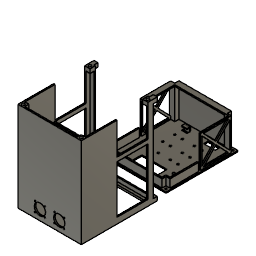
all 600 w (Autodesk Fusion 360 design; units mm, degrees)
part number: 2026-06-05-11-29-00-149
Autodesk Fusion 360 part; units mm, degrees
note: some values were not read from the file. Set by a fixed rule: which sketch regions a step uses.
(part 1 of 2)
sketch "Sketch3" plane through (0, 0, 0) normal (0, 0, 1) x (1, 0, 0)
  line L0 (79.125, -47) -> (-79.125, -47)
  line L1 (-79.125, -47) -> (-79.125, 47)
  line L2 (-79.125, 47) -> (79.125, 47)
  line L3 (79.125, 47) -> (79.125, -47)
  line L4 (79.125, -47) -> (-79.125, 47) construction
  line L5 (-79.125, -47) -> (79.125, 47) construction
  dimension "d3" = 94
  dimension "d4" = 158.25
  constraint horizontal L0
  constraint perpendicular L0 L1
  constraint parallel L0 L2
  constraint parallel L1 L3
  constraint coincident L4 origin
  constraint coincident L5 origin
  measures "d3" distance of L0.end L1.end
  measures "d4" distance of L1.end L2.end
extrude "Extrude1" add sketch "Sketch3" along normal blind 15 makes body 1
sketch "Sketch4" plane through (0, 0, 15) normal (0, 0, 1) x (-1, 0, 0)
  line L0 (-79.125, -47) -> (79.125, -47)
  line L1 (79.125, -47) -> (79.125, 47)
  line L2 (79.125, 47) -> (-79.125, 47)
  line L3 (-79.125, 47) -> (-79.125, -47)
  line L4 (-75.625, 43.5) -> (75.625, 43.5)
  line L5 (75.625, 43.5) -> (75.625, -43.5)
  line L6 (75.625, -43.5) -> (-75.625, -43.5)
  line L7 (-75.625, -43.5) -> (-75.625, 43.5)
  dimension "d7" = 3.5
  dimension "d9" = 3.5
  dimension "d10" = 3.5
  dimension "d11" = 3.5
  constraint horizontal L4
  constraint perpendicular L4 L5
  constraint parallel L4 L6
  constraint parallel L5 L7
  measures "d7" distance of L2 L4
  measures "d9" distance of L3 L7
  measures "d10" distance of L1 L5
  measures "d11" distance of L0 L6
extrude "Extrude2" cut sketch "Sketch4" against normal blind 10 contours L4 L5 L6 L7 bodies 1
sketch "Sketch5" plane through (0, 0, 5) normal (0, 0, 1) x (-1, 0, 0)
  line L0 (-75.625, -43.5) -> (75.625, -43.5)
  line L1 (75.625, -43.5) -> (75.625, 43.5)
  line L2 (75.625, 43.5) -> (-75.625, 43.5)
  line L3 (-75.625, 43.5) -> (-75.625, -43.5)
  line L4 (-69.125, 37) -> (69.125, 37)
  line L5 (69.125, 37) -> (69.125, -37)
  line L6 (69.125, -37) -> (-69.125, -37)
  line L7 (-69.125, -37) -> (-69.125, 37)
  dimension "d14" = 6.5
  dimension "d15" = 6.5
  dimension "d16" = 6.5
  dimension "d17" = 6.5
  constraint horizontal L4
  constraint perpendicular L4 L5
  constraint parallel L4 L6
  constraint parallel L5 L7
  measures "d14" distance of L3 L7
  measures "d15" distance of L2 L4
  measures "d16" distance of L0 L6
  measures "d17" distance of L1 L5
extrude "Extrude3" cut sketch "Sketch5" against normal blind 5 contours L4 L5 L6 L7 bodies 1
sketch "Sketch6" plane through (0, -47, 0) normal (0, -1, 0) x (1, 0, 0)
  line L0 (-79.125, 0) -> (79.125, 0)
  line L1 (79.125, 0) -> (79.125, 15)
  line L2 (79.125, 15) -> (-79.125, 15)
  line L3 (-79.125, 15) -> (-79.125, 0)
  line L4 (-79.125, 5) -> (79.125, 5)
  line L5 (79.125, 5) -> (79.125, 0)
  line L6 (79.125, 0) -> (-79.125, 0)
  line L7 (-79.125, 0) -> (-79.125, 5)
  dimension "d20" = 5
  constraint horizontal L4
  constraint vertical L5
  constraint horizontal L6
  constraint vertical L7
  constraint coincident L0.end L1.start
  constraint coincident L3 L4.start
  measures "d20" distance of L4 L6
extrude "Extrude4" add sketch "Sketch6" along normal blind 86 contours L0 L1 L3 L4 L5 L6 L7 bodies 1
sketch "Sketch7" plane through (0, 0, 5) normal (0, 0, 1) x (-1, 0, 0)
  line L0 (-79.125, 47) -> (79.125, 47)
  line L1 (79.125, 47) -> (79.125, 133)
  line L2 (79.125, 133) -> (-79.125, 133)
  line L3 (-79.125, 133) -> (-79.125, 47)
  line L4 (79.125, 47) -> (75.625, 47)
  line L5 (75.625, 47) -> (75.625, 129.5)
  line L6 (75.625, 133) -> (79.125, 133)
  line L7 (79.125, 133) -> (79.125, 47)
  line L8 (79.125, 133) -> (-79.125, 133)
  line L9 (-79.125, 133) -> (-79.125, 118.5)
  line L10 (-75.625, 129.5) -> (75.625, 129.5)
  line L11 (79.125, 118.5) -> (79.125, 133)
  line L12 (-79.125, 133) -> (-75.625, 133)
  line L13 (-75.625, 129.5) -> (-75.625, 47)
  line L14 (-75.625, 47) -> (-79.125, 47)
  line L15 (-79.125, 47) -> (-79.125, 133)
  dimension "d23" = 3.5
  dimension "d24" = 3.5
  dimension "d25" = 3.5
  constraint horizontal L4
  constraint vertical L5
  constraint horizontal L6
  constraint vertical L7
  constraint coincident L2 L6.start
  constraint coincident L0.end L1.start
  constraint horizontal L8
  constraint vertical L9
  constraint horizontal L10
  constraint vertical L11
  constraint coincident L3 L9.end
  constraint coincident L1.end L2.start
  constraint horizontal L12
  constraint vertical L13
  constraint horizontal L14
  constraint vertical L15
  constraint coincident L0 L13.end
  measures "d23" distance of L5 L7
  measures "d24" distance of L8 L10
  measures "d25" distance of L13 L15
extrude "Extrude5" add sketch "Sketch7" along normal blind 10 contours L0 L1 L2 L3 L4 L5 L6 L7 L8 L9 L10 L11 L12 L13 L14 L15 bodies 1
sketch "Sketch8" plane through (0, 0, 15) normal (0, 0, 1) x (-1, 0, 0)
  line L0 (75.625, 47) -> (-75.625, 47)
  line L1 (-75.625, 47) -> (-75.625, 129.5)
  line L2 (-75.625, 129.5) -> (75.625, 129.5)
  line L3 (75.625, 129.5) -> (75.625, 47)
  line L4 (75.625, 43.5) -> (75.625, -43.5)
  line L5 (75.625, -43.5) -> (-75.625, -43.5)
  line L6 (-75.625, -43.5) -> (-75.625, 43.5)
  line L7 (-75.625, 43.5) -> (75.625, 43.5)
  line L8 (79.125, -47) -> (79.125, 133)
  line L9 (79.125, 133) -> (-79.125, 133)
  line L10 (-79.125, 133) -> (-79.125, -47)
  line L11 (-79.125, -47) -> (79.125, -47)
  line L12 (75.625, 43.5) -> (79.125, 43.5)
  line L13 (-75.625, 43.5) -> (-79.125, 43.5)
  constraint coincident L4.start L7.end
  constraint coincident L8 L12.end
  constraint perpendicular L8 L12
  constraint coincident L6.end L7.start
  constraint coincident L10 L13.end
  constraint perpendicular L10 L13
extrude "Extrude6" add sketch "Sketch8" along normal blind 130 contours L7 L8 L9 L10 L12 L13 bodies 1
sketch "Sketch9" plane through (0, 0, 15) normal (0, 0, 1) x (-1, 0, 0)
  line L0 (79.125, 43.5) -> (75.625, 43.5)
  line L1 (75.625, 43.5) -> (75.625, -43.5)
  line L2 (75.625, -43.5) -> (-75.625, -43.5)
  line L3 (-75.625, -43.5) -> (-75.625, 43.5)
  line L4 (-75.625, 43.5) -> (-79.125, 43.5)
  line L5 (-79.125, 43.5) -> (-79.125, -47)
  line L6 (-79.125, -47) -> (79.125, -47)
  line L7 (79.125, -47) -> (79.125, 43.5)
  line L8 (-79.125, -47) -> (-75.625, -47)
  line L9 (-75.625, -47) -> (-75.625, -43.5)
  line L10 (-75.625, -43.5) -> (-79.125, -43.5)
  line L11 (-79.125, -43.5) -> (-79.125, -47)
  line L12 (75.625, -43.5) -> (79.125, -43.5)
  line L13 (79.125, -43.5) -> (79.125, -47)
  line L14 (79.125, -47) -> (75.625, -47)
  line L15 (75.625, -47) -> (75.625, -43.5)
  constraint horizontal L8
  constraint vertical L9
  constraint horizontal L10
  constraint vertical L11
  constraint coincident L2.end L3.start
  constraint coincident L5.end L6.start
  constraint horizontal L12
  constraint vertical L13
  constraint horizontal L14
  constraint vertical L15
  constraint coincident L6.end L7.start
  constraint coincident L1.end L2.start
extrude "Extrude7" add sketch "Sketch9" along normal blind 130 contours L6 L7 L12 L13 L14 L15 | L5 L6 L8 L9 L10 L11 bodies 1
extrude "Extrude8" add 1 faces at (75.625, 45.8333, 58.3333) along direction (-1, 0, 0) blind 10 on bodies 1 bodies 1
extrude "Extrude9" add 1 faces at (-75.625, 45.8333, 58.3333) along direction (1, 0, 0) blind 10 on bodies 1 bodies 1
sketch "Sketch10" plane through (0, 43.5, 0) normal (0, -1, 0) x (1, 0, 0)
  line L0 (-79.125, 15) -> (-75.625, 15)
  line L1 (-75.625, 15) -> (-75.625, 5)
  line L2 (-75.625, 5) -> (75.625, 5)
  line L3 (75.625, 5) -> (75.625, 15)
  line L4 (75.625, 15) -> (79.125, 15)
  line L5 (79.125, 15) -> (79.125, 145)
  line L6 (79.125, 145) -> (65.625, 145)
  line L7 (65.625, 145) -> (65.625, 15)
  line L8 (65.625, 15) -> (-65.625, 15)
  line L9 (-65.625, 15) -> (-65.625, 145)
  line L10 (-65.625, 145) -> (-79.125, 145)
  line L11 (-79.125, 145) -> (-79.125, 15)
  line L12 (-79.125, 145) -> (-75.625, 145)
  line L13 (-75.625, 145) -> (-75.625, 15)
  line L14 (-75.625, 15) -> (-79.125, 15)
  line L15 (-79.125, 15) -> (-79.125, 145)
  dimension "d36" = 3.5
  dimension "d37" = 130
  constraint horizontal L12
  constraint vertical L13
  constraint horizontal L14
  constraint vertical L15
  constraint coincident L10.end L11.start
  measures "d36" distance of L10.end L12.end
  measures "d37" distance of L10.end L0.start
extrude "Extrude10" add sketch "Sketch10" along normal blind 10 contours L0 L10 L11 L12 L13 L14 L15 bodies 1
sketch "Sketch11" plane through (0, 43.5, 0) normal (0, -1, 0) x (1, 0, 0)
  line L0 (-75.625, 145) -> (-75.625, 5)
  line L1 (-75.625, 5) -> (75.625, 5)
  line L2 (75.625, 5) -> (75.625, 15)
  line L3 (75.625, 15) -> (79.125, 15)
  line L4 (79.125, 15) -> (79.125, 145)
  line L5 (79.125, 145) -> (65.625, 145)
  line L6 (65.625, 145) -> (65.625, 15)
  line L7 (65.625, 15) -> (-65.625, 15)
  line L8 (-65.625, 15) -> (-65.625, 145)
  line L9 (-65.625, 145) -> (-75.625, 145)
  line L10 (79.125, 15) -> (75.625, 15)
  line L11 (75.625, 15) -> (75.625, 145)
  line L12 (75.625, 145) -> (79.125, 145)
  line L13 (79.125, 145) -> (79.125, 15)
  constraint perpendicular L10 L11
  constraint parallel L10 L12
  constraint parallel L11 L13
  constraint coincident L2.end L3.start
  constraint perpendicular L2 L10
  constraint coincident L3.end L4.start
extrude "Extrude11" add sketch "Sketch11" along normal blind 10 contours L3 L4 L5 L10 L11 L12 L13 bodies 1
sketch "Sketch13" plane through (0, 33.5, 0) normal (0, -1, 0) x (1, 0, 0)
  line L0 (-79.125, 15) -> (-75.625, 15)
  line L1 (-75.625, 15) -> (-75.625, 145)
  line L2 (-75.625, 145) -> (-79.125, 145)
  line L3 (-79.125, 145) -> (-79.125, 15)
  line L4 (-79.125, 145) -> (-75.625, 145)
  line L5 (-75.625, 145) -> (-75.625, 135)
  line L6 (-75.625, 135) -> (-79.125, 135)
  line L7 (-79.125, 135) -> (-79.125, 145)
  dimension "d45" = 10
  constraint horizontal L4
  constraint vertical L5
  constraint horizontal L6
  constraint vertical L7
  constraint coincident L2.end L3.start
  measures "d45" distance of L2.end L6.end
extrude "Extrude13" add sketch "Sketch13" along normal blind 77 contours L1 L2 L3 L4 L5 L6 L7 bodies 1
sketch "Sketch14" plane through (0, 33.5, 0) normal (0, -1, 0) x (1, 0, 0)
  line L0 (79.125, 145) -> (75.625, 145)
  line L1 (75.625, 145) -> (75.625, 15)
  line L2 (75.625, 15) -> (79.125, 15)
  line L3 (79.125, 15) -> (79.125, 145)
  line L4 (75.625, 145) -> (79.125, 145)
  line L5 (79.125, 145) -> (79.125, 135)
  line L6 (79.125, 135) -> (75.625, 135)
  line L7 (75.625, 135) -> (75.625, 145)
  dimension "d48" = 10
  constraint horizontal L4
  constraint vertical L5
  constraint horizontal L6
  constraint vertical L7
  constraint coincident L0.end L1.start
  measures "d48" distance of L0.end L6.end
extrude "Extrude14" add sketch "Sketch14" along normal blind 77 contours L0 L1 L3 L4 L5 L6 L7 bodies 1
sketch "Sketch15" plane through (0, 47, 0) normal (0, 1, 0) x (-1, 0, 0)
  line L0 (65.625, 145) -> (65.625, 15)
  line L1 (65.625, 15) -> (-65.625, 15)
  line L2 (-65.625, 15) -> (-65.625, 145)
  line L3 (79.125, 145) -> (65.625, 145)
  line L4 (-79.125, 145) -> (-79.125, 0)
  line L5 (-79.125, 0) -> (79.125, 0)
  line L6 (79.125, 0) -> (79.125, 145)
  line L7 (79.125, 0) -> (69.125, 0)
  line L8 (69.125, 0) -> (69.125, 10)
  line L9 (69.125, 10) -> (79.125, 10)
  line L10 (79.125, 10) -> (79.125, 0)
  line L11 (-65.625, 145) -> (-79.125, 145)
  dimension "d51" = 10
  dimension "d52" = 10
  constraint horizontal L7
  constraint vertical L8
  constraint horizontal L9
  constraint vertical L10
  constraint coincident L5.end L6.start
  measures "d51" distance of L5.end L7.end
  measures "d52" distance of L5.end L9.end
extrude "Extrude15" add sketch "Sketch15" along normal blind 10 contours L5 L6 L7 L8 L9 L10 bodies 1
sketch "Sketch16" plane through (0, 47, 0) normal (0, 1, 0) x (-1, 0, 0)
  line L0 (69.125, 0) -> (69.125, 10)
  line L1 (69.125, 10) -> (79.125, 10)
  line L2 (79.125, 10) -> (79.125, 145)
  line L3 (79.125, 145) -> (65.625, 145)
  line L4 (-79.125, 145) -> (-79.125, 0)
  line L5 (-79.125, 0) -> (69.125, 0)
  line L6 (65.625, 145) -> (65.625, 15)
  line L7 (65.625, 15) -> (-65.625, 15)
  line L8 (-65.625, 15) -> (-65.625, 145)
  line L9 (-79.125, 0) -> (-69.125, 0)
  line L10 (-69.125, 0) -> (-69.125, 10)
  line L11 (-69.125, 10) -> (-79.125, 10)
  line L12 (-79.125, 10) -> (-79.125, 0)
  line L13 (-65.625, 145) -> (-79.125, 145)
  dimension "d55" = 10
  dimension "d56" = 10
  constraint horizontal L9
  constraint vertical L10
  constraint horizontal L11
  constraint vertical L12
  constraint coincident L4.end L5.start
  measures "d55" distance of L4.end L9.end
  measures "d56" distance of L4.end L11.end
extrude "Extrude16" add sketch "Sketch16" along normal blind 10 contours L4 L5 L9 L10 L11 L12 bodies 1
move_body "Move1" bodies 1 to x (1, 0, 0) y (0, 1, 0) z (0, 0, 1) at (235.1887, 10.9866, 0)
sketch "Sketch18" plane through (0, 0, 0) normal (0, 0, 1) x (1, 0, 0)
  line L0 (79.125, -90) -> (-79.125, -90)
  line L1 (-79.125, -90) -> (-79.125, 90)
  line L2 (-79.125, 90) -> (79.125, 90)
  line L3 (79.125, 90) -> (79.125, -90)
  line L4 (79.125, -90) -> (-79.125, 90) construction
  line L5 (-79.125, -90) -> (79.125, 90) construction
  dimension "d63" = 158.25
  dimension "d64" = 180
  constraint horizontal L0
  constraint perpendicular L0 L1
  constraint parallel L0 L2
  constraint parallel L1 L3
  constraint coincident L4 origin
  constraint coincident L5 origin
  measures "d63" distance of L1.end L2.end
  measures "d64" distance of L0.end L1.end
extrude "Extrude17" add sketch "Sketch18" along normal blind 3 separate body makes body 2
sketch "Sketch19" plane through (0, 0, 3) normal (0, 0, 1) x (-1, 0, 0)
  line L0 (-79.125, -90) -> (79.125, -90)
  line L1 (79.125, -90) -> (79.125, 90)
  line L2 (79.125, 90) -> (-79.125, 90)
  line L3 (-79.125, 90) -> (-79.125, -90)
  line L4 (-31.5, 81) -> (31.5, 81)
  line L5 (31.5, 81) -> (31.5, 40)
  line L6 (31.5, 40) -> (-31.5, 40)
  line L7 (-31.5, 40) -> (-31.5, 81)
  dimension "d67" = 63
  dimension "d68" = 41
  dimension "d329" = 9
  dimension "d367" = 47.625
  constraint horizontal L4
  constraint vertical L5
  constraint horizontal L6
  constraint vertical L7
  measures "d67" distance of L4.start L4.end
  measures "d68" distance of L4.start L6.end
  measures "d329" distance of L2 L4
  measures "d367" distance of L3 L7
extrude "Extrude18" cut sketch "Sketch19" against normal blind 3 contours L4 L5 L6 L7 bodies 2
sketch "Sketch20" plane through (0, 0, 3) normal (0, 0, 1) x (-1, 0, 0)
  line L0 (31.5, 81) -> (31.5, 40)
  line L1 (31.5, 40) -> (-31.5, 40)
  line L2 (-31.5, 40) -> (-31.5, 81)
  line L3 (-31.5, 81) -> (31.5, 81)
  line L4 (-79.125, -90) -> (79.125, -90)
  line L5 (79.125, -90) -> (79.125, 90)
  line L6 (79.125, 90) -> (-79.125, 90)
  line L7 (-79.125, 90) -> (-79.125, -90)
  circle A0 centre (-15, 15) radius 2.5
  circle A1 centre (-34, 15) radius 2.5
  circle A2 centre (-34, -15) radius 2.5
  circle A3 centre (-15, -15) radius 2.5
  circle A4 centre (-15, -45) radius 2.5
  circle A5 centre (-34, -45) radius 2.5
  line L8 (-34, 15) -> (-15, 15)
  line L9 (-15, 15) -> (-15, -15)
  line L10 (-15, -15) -> (-34, -15)
  line L11 (-34, -15) -> (-34, 15)
  line L12 (-15, -45) -> (-15, -15)
  line L13 (-15, -45) -> (-34, -45)
  line L14 (-34, -15) -> (-34, -45)
  circle A6 centre (15, 15) radius 2.5
  circle A7 centre (34, 15) radius 2.5
  circle A8 centre (15, -15) radius 2.5
  circle A9 centre (34, -15) radius 2.5
  circle A10 centre (15, -45) radius 2.5
  circle A11 centre (34, -45) radius 2.5
  line L15 (15, 15) -> (34, 15)
  line L16 (34, 15) -> (34, -15)
  line L17 (34, -15) -> (15, -15)
  line L18 (15, -15) -> (15, 15)
  line L19 (15, -15) -> (15, -45)
  line L20 (15, -45) -> (34, -45)
  line L21 (34, -45) -> (34, -15)
  line L22 (15, 15) -> (-15, 15)
  line L23 (-15, -15) -> (15, -15)
  line L24 (15, -45) -> (-15, -45)
  dimension "d71" = 5
  dimension "d72" = 5
  dimension "d73" = 5
  dimension "d74" = 5
  dimension "d75" = 5
  dimension "d76" = 5
  dimension "d77" = 19
  dimension "d78" = 75
  dimension "d79" = 75
  dimension "d80" = 30
  dimension "d353" = 5
  dimension "d354" = 5
  dimension "d355" = 5
  dimension "d356" = 5
  dimension "d357" = 5
  dimension "d358" = 5
  dimension "d359" = 30
  dimension "d360" = 30
  dimension "d361" = 19
  dimension "d362" = 30
  dimension "d363" = 30
  dimension "d364" = 75
  dimension "d365" = 30
  dimension "d366" = 45.125
  constraint coincident A1.centre L8.start
  constraint coincident A0.centre L8.end
  constraint coincident A3.centre L9.end
  constraint coincident A2.centre L10.end
  constraint coincident A5.centre L13.end
  constraint coincident A4.centre L12.start
  constraint parallel L8 L10
  constraint parallel L10 L13
  constraint equal L8 L10
  constraint equal L10 L13
  constraint equal L11 L12
  constraint perpendicular L10 L11
  constraint perpendicular L10 L14
  constraint coincident A6.centre L15.start
  constraint coincident A7.centre L15.end
  constraint coincident A9.centre L16.end
  constraint coincident A8.centre L17.end
  constraint vertical L18
  constraint coincident A10.centre L19.end
  constraint coincident A11.centre L20.end
  constraint parallel L6 L15
  constraint equal L15 L17
  constraint equal L17 L20
  constraint perpendicular L17 L19
  measures "d71" diameter of A0
  measures "d72" diameter of A1
  measures "d73" diameter of A2
  measures "d74" diameter of A3
  measures "d75" diameter of A4
  measures "d76" diameter of A5
  measures "d77" horizontal distance of A0.centre A1.centre
  measures "d78" distance of L6 A1.centre
  measures "d79" distance of L6 A0.centre
  measures "d80" distance of A1.centre A2.centre
  measures "d353" diameter of A6
  measures "d354" diameter of A7
  measures "d355" diameter of A8
  measures "d356" diameter of A9
  measures "d358" diameter of A11
  measures "d359" vertical distance of A8.centre A10.centre
  measures "d360" distance of A6.centre A8.centre
  measures "d361" horizontal distance of A6.centre A7.centre
  measures "d362" vertical distance of A7.centre A9.centre
  measures "d363" vertical distance of A9.centre A11.centre
  measures "d364" distance of L6 A6.centre
  measures "d365" distance of A0.centre A6.centre
  measures "d366" distance of L7 L11
extrude "Extrude19" cut sketch "Sketch20" against normal blind 3 contours A0 L8 L22 | A0 L9 L22 | A0 L8 L9 | A6 L18 L22 | A6 L15 L22 | A1 L8 L11 | A1 L8 L11 | A3 L9 L10 | A3 L9 L23 | A6 L15 L18 | A3 L12 L23 | A3 L10 L12 | A7 L15 L16 | A7 L15 L16 | A8 L18 L23 | A8 L17 L18 | A2 L11 L14 | A2 L10 L11 | A8 L19 L23 | A2 L10 L14 | A8 L17 L19 | A4 L12 L13 | A4 L12 L24 | A9 L16 L17 | A9 L16 L21 | A9 L17 L21 | A5 L13 L14 | A5 L13 L14 | A4 L13 L24 | A10 L19 L24 | A10 L19 L20 | A10 L20 L24 | A11 L20 L21 | A11 L20 L21 bodies 2
sketch "Sketch21" plane through (0, 0, 3) normal (0, 0, 1) x (-1, 0, 0)
  line L0 (-79.125, -90) -> (79.125, -90)
  line L1 (79.125, -90) -> (79.125, 90)
  line L2 (79.125, 90) -> (-79.125, 90)
  line L3 (-79.125, 90) -> (-79.125, -90)
  line L4 (31.5, 81) -> (31.5, 40)
  line L5 (31.5, 40) -> (-31.5, 40)
  line L6 (-31.5, 40) -> (-31.5, 81)
  line L7 (-31.5, 81) -> (31.5, 81)
  circle A0 centre (-15, -45) radius 2.5
  circle A1 centre (-15, 15) radius 2.5
  circle A2 centre (-15, -15) radius 2.5
  circle A3 centre (-34, -45) radius 2.5
  circle A4 centre (-34, 15) radius 2.5
  circle A5 centre (-34, -15) radius 2.5
  circle A6 centre (49.125, 40) radius 3.5
  circle A7 centre (34, -45) radius 2.5
  circle A8 centre (15, 15) radius 2.5
  circle A9 centre (15, -15) radius 2.5
  circle A10 centre (15, -45) radius 2.5
  circle A11 centre (34, 15) radius 2.5
  circle A12 centre (34, -15) radius 2.5
  dimension "d84" = 7
  dimension "d368" = 50
  dimension "d369" = 30
  measures "d84" diameter of A6
  measures "d368" distance of L2 A6.centre
  measures "d369" distance of L1 A6.centre
extrude "Extrude20" cut sketch "Sketch21" against normal blind 3 contours A6 bodies 2
sketch "Sketch22" plane through (0, 0, 3) normal (0, 0, 1) x (-1, 0, 0)
  circle A0 centre (-34, -15) radius 2.5
  circle A1 centre (-34, -45) radius 2.5
  circle A2 centre (-15, -15) radius 2.5
  circle A3 centre (-15, 15) radius 2.5
  circle A4 centre (-15, -45) radius 2.5
  line L0 (31.5, 81) -> (31.5, 40)
  line L1 (31.5, 40) -> (-31.5, 40)
  line L2 (-31.5, 40) -> (-31.5, 81)
  line L3 (-31.5, 81) -> (31.5, 81)
  line L4 (-79.125, -90) -> (79.125, -90)
  line L5 (79.125, -90) -> (79.125, 90)
  line L6 (79.125, 90) -> (-79.125, 90)
  line L7 (-79.125, 90) -> (-79.125, -90)
  line L8 (21.4933, -61.9167) -> (50.1933, -61.9167)
  line L9 (50.1933, -61.9167) -> (50.1933, -72.9167)
  line L10 (50.1933, -72.9167) -> (21.4933, -72.9167)
  line L11 (21.4933, -72.9167) -> (21.4933, -61.9167)
  circle A5 centre (-34, 15) radius 2.5
  circle A6 centre (34, -15) radius 2.5
  circle A7 centre (34, 15) radius 2.5
  circle A8 centre (15, -45) radius 2.5
  circle A9 centre (15, -15) radius 2.5
  circle A10 centre (15, 15) radius 2.5
  circle A11 centre (34, -45) radius 2.5
  circle A12 centre (49.125, 40) radius 3.5
  dimension "d87" = 28.7
  dimension "d88" = 11
  constraint horizontal L8
  constraint vertical L9
  constraint horizontal L10
  constraint vertical L11
  measures "d87" distance of L8.start L8.end
  measures "d88" distance of L8.start L10.end
extrude "Extrude21" cut sketch "Sketch22" against normal blind 3 contours L8 L9 L10 L11 bodies 2
move_body "Move3" bodies 2 to x (-1, 0, 0) y (0, 1, 0) z (0, 0, -1) at (-44.4015, 0, 3)
sketch "Sketch25" plane through (0, 0, 3) normal (0, 0, 1) x (-1, 0, 0)
  line L0 (-5.7917, -72.9167) -> (-5.7917, -61.9167)
  line L1 (-5.7917, -61.9167) -> (22.9083, -61.9167)
  line L2 (22.9083, -61.9167) -> (22.9083, -72.9167)
  line L3 (22.9083, -72.9167) -> (-5.7917, -72.9167)
  circle A0 centre (78.4015, -15) radius 2.5
  circle A1 centre (78.4015, -45) radius 2.5
  circle A2 centre (59.4015, -15) radius 2.5
  circle A3 centre (59.4015, 15) radius 2.5
  circle A4 centre (59.4015, -45) radius 2.5
  line L4 (12.9015, 40) -> (12.9015, 81)
  line L5 (12.9015, 81) -> (75.9015, 81)
  line L6 (75.9015, 81) -> (75.9015, 40)
  line L7 (75.9015, 40) -> (12.9015, 40)
  line L8 (-34.7235, -90) -> (123.5265, -90)
  line L9 (123.5265, -90) -> (123.5265, 90)
  line L10 (123.5265, 90) -> (-34.7235, 90)
  line L11 (-34.7235, 90) -> (-34.7235, -90)
  line L12 (-21.2235, -87) -> (110.0265, -87)
  line L13 (106.5265, -83.5) -> (-17.7235, -83.5)
  line L14 (116.5265, -73) -> (116.5265, 0)
  line L15 (116.5265, 0) -> (120.0265, 0)
  line L16 (-27.7235, -73) -> (-27.7235, 0)
  line L17 (-27.7235, 0) -> (-31.2235, 0)
  line L18 (-31.2235, 0) -> (-31.2235, -76.5)
  line L19 (-21.2235, -76.5) -> (-31.2235, -76.5)
  line L20 (-17.7235, -76.5) -> (-17.7235, -73)
  line L21 (-17.7235, -73) -> (-27.7235, -73)
  line L22 (-17.7235, -76.5) -> (-17.7235, -83.5)
  line L23 (120.0265, 0) -> (120.0265, -76.5)
  line L24 (110.0265, -76.5) -> (110.0265, -83.5)
  line L25 (110.0265, -83.5) -> (110.0265, -87)
  line L26 (116.5265, -73) -> (106.5265, -73)
  line L27 (106.5265, -83.5) -> (106.5265, -73)
  line L28 (110.0265, -76.5) -> (120.0265, -76.5)
  line L29 (-21.2235, -76.5) -> (-21.2235, -87)
  circle A5 centre (78.4015, 15) radius 2.5
  circle A6 centre (10.4015, -45) radius 2.5
  circle A7 centre (29.4015, 15) radius 2.5
  circle A8 centre (29.4015, -15) radius 2.5
  circle A9 centre (29.4015, -45) radius 2.5
  circle A10 centre (10.4015, 15) radius 2.5
  circle A11 centre (10.4015, -15) radius 2.5
  circle A12 centre (-4.7235, 40) radius 3.5
  dimension "d101" = 3
  dimension "d105" = 3.5
  dimension "d107" = 3.5
  constraint horizontal L12
  constraint horizontal L13
  constraint vertical L14
  constraint horizontal L15
  constraint vertical L16
  constraint horizontal L17
  constraint vertical L18
  constraint horizontal L19
  constraint vertical L20
  constraint horizontal L21
  constraint perpendicular L13 L22
  constraint perpendicular L15 L23
  constraint vertical L24
  constraint perpendicular L26 L27
  constraint perpendicular L23 L28
  constraint perpendicular L19 L29
  measures "d101" distance of L8 L12
  measures "d105" distance of L14.end L15.end
  measures "d107" distance of L16.end L17.end
extrude "Extrude23" add sketch "Sketch25" along normal blind 80 contours L12 L13 L14 L15 L16 L17 L18 L19 L20 L21 L22 L23 L24 L25 L26 L27 L28 L29 bodies 2
sketch "Sketch26" plane through (0, 83.5, 0) normal (0, -1, 0) x (1, 0, 0)
  line L0 (-106.5265, 3) -> (17.7235, 3)
  line L1 (17.7235, 83) -> (-106.5265, 83)
  line L2 (-106.5265, 83) -> (17.7235, 83)
  line L3 (17.7235, 83) -> (17.7235, 79.5)
  line L4 (17.7235, 79.5) -> (-106.5265, 79.5)
  line L5 (-106.5265, 79.5) -> (-106.5265, 83)
  line L6 (17.7235, 3) -> (17.7235, 83)
  line L7 (-106.5265, 83) -> (-106.5265, 3)
  dimension "d108" = 3.5
  dimension "d187" = 124.25
  constraint horizontal L2
  constraint vertical L3
  constraint horizontal L4
  constraint vertical L5
  constraint coincident L1.end L2.start
  measures "d108" distance of L2 L4
  measures "d187" distance of L3 L5
extrude "Extrude24" add sketch "Sketch26" along normal blind 10.5 contours L1 L2 L3 L4 L5 L6 L7 bodies 2
sketch "Sketch27" plane through (-116.5265, 0, 0) normal (1, 0, 0) x (0, 1, 0)
  line L0 (73, 83) -> (0, 83)
  line L1 (0, 83) -> (0, 3)
  line L2 (0, 3) -> (73, 3)
  line L3 (0, 83) -> (73, 83)
  line L4 (73, 83) -> (73, 79.5)
  line L5 (73, 79.5) -> (0, 79.5)
  line L6 (0, 79.5) -> (0, 83)
  line L7 (73, 3) -> (73, 83)
  dimension "d188" = 73
  dimension "d420" = 3.5
  constraint horizontal L3
  constraint vertical L4
  constraint horizontal L5
  constraint vertical L6
  constraint coincident L0.end L1.start
  measures "d188" distance of L0.end L0.start
  measures "d420" distance of L3 L5
extrude "Extrude25" add sketch "Sketch27" along normal blind 10 contours L0 L1 L3 L4 L5 L6 L7 bodies 2
sketch "Sketch30" plane through (0, 0, 145) normal (0, 0, 1) x (-1, 0, 0)
  line L0 (-314.3137, 122.0134) -> (-314.3137, -57.9866)
  line L1 (-314.3137, -57.9866) -> (-300.8137, -57.9866)
  line L2 (-156.0637, -57.9866) -> (-156.0637, 122.0134)
  line L3 (-156.0637, 122.0134) -> (-314.3137, 122.0134)
  line L4 (-310.8137, 118.5134) -> (-159.5637, 118.5134)
  line L5 (-159.5637, 118.5134) -> (-159.5637, 36.0134)
  line L6 (-159.5637, 36.0134) -> (-310.8137, 36.0134)
  line L7 (-310.8137, 36.0134) -> (-310.8137, 118.5134)
  line L8 (-310.8137, -54.4866) -> (-310.8137, 32.5134)
  line L9 (-310.8137, 32.5134) -> (-159.5637, 32.5134)
  line L10 (-159.5637, 32.5134) -> (-159.5637, -54.4866)
  line L11 (-300.8137, -54.4866) -> (-310.8137, -54.4866)
  line L12 (-159.5637, 36.0134) -> (-159.5637, 32.5134)
  line L13 (-159.5637, 32.5134) -> (-156.0637, 32.5134)
  line L14 (-310.8137, 36.0134) -> (-310.8137, 32.5134)
  line L15 (-314.3137, 32.5134) -> (-310.8137, 32.5134)
  line L16 (-300.8137, -57.9866) -> (-300.8137, -54.4866)
  line L17 (-159.5637, -54.4866) -> (-169.5637, -54.4866)
  line L18 (-169.5637, -54.4866) -> (-169.5637, -57.9866)
  line L19 (-169.5637, -57.9866) -> (-156.0637, -57.9866)
  constraint coincident L5.end L6.start
  constraint coincident L9.end L10.start
  constraint coincident L2 L13.end
  constraint perpendicular L2 L13
  constraint coincident L6.end L7.start
  constraint coincident L8.end L9.start
  constraint coincident L0 L15.start
  constraint perpendicular L8 L15
extrude "Extrude27" add sketch "Sketch30" along normal blind 80 contours L0 L2 L3 L4 L5 L7 L12 L13 L14 L15 bodies 1
sketch "Sketch31" plane through (0, 0, 3) normal (0, 0, 1) x (-1, 0, 0)
  line L0 (-34.7235, -90) -> (123.5265, -90)
  line L1 (123.5265, -90) -> (123.5265, 90)
  line L2 (123.5265, 90) -> (-34.7235, 90)
  line L3 (-34.7235, 90) -> (-34.7235, -90)
  line L4 (12.9015, 40) -> (12.9015, 81)
  line L5 (12.9015, 81) -> (75.9015, 81)
  line L6 (75.9015, 81) -> (75.9015, 40)
  line L7 (75.9015, 40) -> (12.9015, 40)
  circle A0 centre (59.4015, -45) radius 2.5
  circle A1 centre (59.4015, 15) radius 2.5
  circle A2 centre (59.4015, -15) radius 2.5
  circle A3 centre (78.4015, -45) radius 2.5
  circle A4 centre (78.4015, -15) radius 2.5
  line L8 (-5.7917, -72.9167) -> (-5.7917, -61.9167)
  line L9 (-5.7917, -61.9167) -> (22.9083, -61.9167)
  line L10 (22.9083, -61.9167) -> (22.9083, -72.9167)
  line L11 (22.9083, -72.9167) -> (-5.7917, -72.9167)
  line L12 (116.5265, -73) -> (116.5265, 0)
  line L13 (116.5265, 0) -> (120.0265, 0)
  line L14 (110.0265, -87) -> (-21.2235, -87)
  line L15 (-31.2235, 0) -> (-27.7235, 0)
  line L16 (-27.7235, 0) -> (-27.7235, -73)
  line L17 (-17.7235, -83.5) -> (106.5265, -83.5)
  line L18 (106.5265, 83) -> (-17.7235, 83)
  line L19 (-27.7235, 73) -> (-27.7235, 5)
  line L20 (-27.7235, 5) -> (-31.2235, 5)
  line L21 (-31.2235, 5) -> (-31.2235, 76.5)
  line L22 (116.5265, 73) -> (116.5265, 5)
  line L23 (120.0265, 5) -> (120.0265, 76.5)
  line L24 (106.5265, -83.5) -> (106.5265, -73)
  line L25 (106.5265, -73) -> (116.5265, -73)
  line L26 (120.0265, 0) -> (120.0265, -76.5)
  line L27 (120.0265, -76.5) -> (110.0265, -76.5)
  line L28 (110.0265, -76.5) -> (110.0265, -87)
  line L29 (-21.2235, -87) -> (-21.2235, -76.5)
  line L30 (-21.2235, -76.5) -> (-31.2235, -76.5)
  line L31 (-31.2235, -76.5) -> (-31.2235, 0)
  line L32 (-27.7235, -73) -> (-17.7235, -73)
  line L33 (-17.7235, -73) -> (-17.7235, -83.5)
  line L34 (110.0265, 76.5) -> (120.0265, 76.5)
  line L35 (106.5265, 83) -> (106.5265, 73)
  line L36 (120.0265, 76.5) -> (110.0265, 76.5)
  line L37 (-21.2235, 86.5) -> (104.0099, 86.5)
  line L38 (116.5265, 73) -> (106.5265, 73)
  line L39 (110.0265, 76.5) -> (110.0265, 86.5)
  line L40 (-21.2235, 86.5) -> (-21.2235, 76.5)
  line L41 (-21.2235, 76.5) -> (-33.7401, 76.5)
  line L42 (-21.2235, 86.5) -> (-17.7235, 86.5)
  line L43 (-21.2235, 76.5) -> (-21.2235, 86.5)
  line L44 (-31.2235, 76.5) -> (-21.2235, 76.5)
  line L45 (-31.2235, 73) -> (-31.2235, 76.5)
  circle A5 centre (78.4015, 15) radius 2.5
  line L46 (-17.7235, 83) -> (-17.7235, 73)
  line L47 (-27.7235, 73) -> (-17.7235, 73)
  line L48 (104.0099, 86.5) -> (110.0265, 86.5)
  circle A6 centre (10.4015, -15) radius 2.5
  circle A7 centre (10.4015, 15) radius 2.5
  circle A8 centre (29.4015, -45) radius 2.5
  circle A9 centre (29.4015, -15) radius 2.5
  circle A10 centre (29.4015, 15) radius 2.5
  circle A11 centre (10.4015, -45) radius 2.5
  circle A12 centre (-4.7235, 40) radius 3.5
  line L49 (120.0265, 5) -> (116.5265, 5)
  dimension "d196" = 3.5
  dimension "d331" = 13.5
  dimension "d332" = 3.5
  dimension "d333" = 13.5
  dimension "d334" = 3.5
  dimension "d337" = 3.5
  dimension "d338" = 3.5
  dimension "d339" = 13.5
  dimension "d340" = 13.5
  dimension "d341" = 3.5
  dimension "d342" = 3.5
  dimension "d344" = 131.25
  dimension "d345" = 3.5
  dimension "d346" = 3.5
  dimension "d347" = 3.5
  dimension "d381" = 5
  dimension "d382" = 5
  constraint vertical L40
  constraint horizontal L41
  constraint horizontal L42
  constraint vertical L43
  constraint horizontal L44
  constraint vertical L45
  constraint perpendicular L46 L47
  constraint perpendicular L39 L48
  constraint perpendicular L22 L49
  measures "d196" distance of L37.start L42.end
  measures "d331" distance of L37 L47
  measures "d332" distance of L41 L47
  measures "d333" distance of L45 L46
  measures "d334" distance of L19 L21
  measures "d337" distance of L18 L37
  measures "d338" distance of L35 L39
  measures "d339" distance of L37 L38
  measures "d340" distance of L23 L35
  measures "d341" distance of L34 L38
  measures "d342" distance of L22 L23
  measures "d344" distance of L39 L40
  measures "d345" distance of L40 L46
  measures "d346" distance of L1 L23
  measures "d347" distance of L2 L37
  measures "d381" distance of L15 L20
  measures "d382" distance of L13 L49
extrude "Extrude28" add sketch "Sketch31" along normal blind 20 contours L18 L19 L20 L21 L22 L23 L34 L35 L36 L37 L38 L39 L40 L41 L42 L43 L44 L45 L46 L47 L48 L49 bodies 2
sketch "Sketch32" plane through (0, 0, 145) normal (0, 0, 1) x (-1, 0, 0)
  line L0 (-156.0637, 32.5134) -> (-159.5637, 32.5134)
  line L1 (-159.5637, 32.5134) -> (-159.5637, -54.4866)
  line L2 (-159.5637, -54.4866) -> (-169.5637, -54.4866)
  line L3 (-310.8137, -54.4866) -> (-310.8137, 32.5134)
  line L4 (-310.8137, 32.5134) -> (-314.3137, 32.5134)
  line L5 (-314.3137, 32.5134) -> (-314.3137, -57.9866)
  line L6 (-169.5637, -57.9866) -> (-156.0637, -57.9866)
  line L7 (-156.0637, -57.9866) -> (-156.0637, 32.5134)
  line L8 (-159.5637, -44.4866) -> (-156.0637, -44.4866)
  line L9 (-169.5637, -54.4866) -> (-169.5637, -57.9866)
  line L10 (-169.5637, -54.4866) -> (-169.5637, -57.9866)
  line L11 (-314.3137, -57.9866) -> (-300.8137, -57.9866)
  line L12 (-300.8137, -57.9866) -> (-300.8137, -54.4866)
  line L13 (-300.8137, -54.4866) -> (-310.8137, -54.4866)
  constraint coincident L1 L8.start
  constraint coincident L7 L8.end
  constraint coincident L2 L9.start
  constraint coincident L6 L9.end
extrude "Extrude31" add sketch "Sketch32" along normal blind 80 contours L1 L2 L6 L7 L8 L9 L10 bodies 1
sketch "Sketch33" plane through (0, 0, 145) normal (0, 0, 1) x (-1, 0, 0)
  line L0 (-310.8137, -54.4866) -> (-310.8137, 32.5134)
  line L1 (-310.8137, -44.4866) -> (-314.3137, -44.4866)
  line L2 (-300.8137, -54.4866) -> (-300.8137, -57.9866)
  line L3 (-300.8137, -54.4866) -> (-310.8137, -54.4866)
  line L4 (-310.8137, 32.5134) -> (-314.3137, 32.5134)
  line L5 (-314.3137, 32.5134) -> (-314.3137, -57.9866)
  line L6 (-314.3137, -57.9866) -> (-300.8137, -57.9866)
  line L7 (-300.8137, -57.9866) -> (-300.8137, -54.4866)
  constraint coincident L0 L1.start
extrude "Extrude30" add sketch "Sketch33" along normal blind 80 contours L0 L1 L2 L3 L5 L6 L7 bodies 1
sketch "Sketch35" plane through (159.5637, 0, 0) normal (1, 0, 0) x (0, 1, 0)
  line L0 (44.4866, 15) -> (-32.5134, 15)
  line L1 (-32.5134, 15) -> (-32.5134, 5)
  line L2 (-32.5134, 5) -> (54.4866, 5)
  line L3 (54.4866, 5) -> (54.4866, 225)
  line L4 (54.4866, 225) -> (44.4866, 225)
  line L5 (44.4866, 225) -> (44.4866, 145)
  line L6 (44.4866, 145) -> (-32.5134, 145)
  line L7 (-32.5134, 145) -> (-32.5134, 135)
  line L8 (-32.5134, 135) -> (44.4866, 135)
  line L9 (44.4866, 135) -> (44.4866, 15)
  line L10 (44.4866, 225) -> (54.4866, 225)
  line L11 (54.4866, 225) -> (54.4866, 215)
  line L12 (54.4866, 215) -> (44.4866, 215)
  line L13 (44.4866, 215) -> (44.4866, 225)
  dimension "d141" = 10
  dimension "d444" = 10
  constraint horizontal L10
  constraint vertical L11
  constraint horizontal L12
  constraint vertical L13
  constraint coincident L4.end L5.start
  measures "d141" distance of L4.end L12.end
  measures "d444" distance of L11 L13
extrude "Extrude32" add sketch "Sketch35" along normal blind 10 contours L3 L4 L5 L10 L11 L12 L13 bodies 1
sketch "Sketch36" plane through (310.8137, 0, 0) normal (-1, 0, 0) x (0, -1, 0)
  line L0 (-54.4866, 225) -> (-54.4866, 5)
  line L1 (-54.4866, 5) -> (32.5134, 5)
  line L2 (32.5134, 5) -> (32.5134, 15)
  line L3 (32.5134, 15) -> (-44.4866, 15)
  line L4 (-44.4866, 15) -> (-44.4866, 135)
  line L5 (-44.4866, 135) -> (32.5134, 135)
  line L6 (32.5134, 135) -> (32.5134, 145)
  line L7 (32.5134, 145) -> (-44.4866, 145)
  line L8 (-44.4866, 145) -> (-44.4866, 225)
  line L9 (-44.4866, 225) -> (-54.4866, 225)
  line L10 (-44.4866, 225) -> (-68.15, 225)
  line L11 (-68.15, 225) -> (-68.15, 215)
  line L12 (-68.15, 215) -> (-44.4866, 215)
  line L13 (-44.4866, 215) -> (-44.4866, 225)
  dimension "d144" = 10
  constraint horizontal L10
  constraint vertical L11
  constraint horizontal L12
  constraint vertical L13
  constraint coincident L8.end L9.start
  measures "d144" distance of L8.end L12.end
extrude "Extrude33" add sketch "Sketch36" along normal blind 10 contours L0 L8 L9 L10 L12 L13 bodies 1
sketch "Sketch37" plane through (0, 57.9866, 0) normal (0, 1, 0) x (-1, 0, 0)
  line L0 (-304.3137, 10) -> (-304.3137, 0)
  line L1 (-304.3137, 0) -> (-166.0637, 0)
  line L2 (-166.0637, 0) -> (-166.0637, 10)
  line L3 (-166.0637, 10) -> (-156.0637, 10)
  line L4 (-156.0637, 10) -> (-156.0637, 225)
  line L5 (-156.0637, 225) -> (-169.5637, 225)
  line L6 (-300.8137, 225) -> (-314.3137, 225)
  line L7 (-314.3137, 225) -> (-314.3137, 10)
  line L8 (-314.3137, 10) -> (-304.3137, 10)
  line L9 (-169.5637, 225) -> (-169.5637, 15)
  line L10 (-169.5637, 15) -> (-300.8137, 15)
  line L11 (-300.8137, 15) -> (-300.8137, 225)
  line L12 (-156.0637, 225) -> (-166.0637, 225)
  line L13 (-166.0637, 225) -> (-166.0637, 215)
  line L14 (-166.0637, 215) -> (-156.0637, 215)
  line L15 (-156.0637, 215) -> (-156.0637, 225)
  dimension "d147" = 10
  dimension "d148" = 10
  constraint horizontal L12
  constraint vertical L13
  constraint horizontal L14
  constraint vertical L15
  constraint coincident L4.end L5.start
  measures "d147" distance of L4.end L12.end
  measures "d148" distance of L4.end L14.end
extrude "Extrude34" add sketch "Sketch37" along normal blind 10 contours L4 L5 L12 L13 L14 L15 bodies 1
sketch "Sketch38" plane through (0, 57.9866, 0) normal (0, 1, 0) x (-1, 0, 0)
  line L0 (-300.8137, 225) -> (-314.3137, 225)
  line L1 (-314.3137, 225) -> (-314.3137, 10)
  line L2 (-314.3137, 10) -> (-304.3137, 10)
  line L3 (-304.3137, 10) -> (-304.3137, 0)
  line L4 (-304.3137, 0) -> (-166.0637, 0)
  line L5 (-166.0637, 0) -> (-166.0637, 10)
  line L6 (-166.0637, 10) -> (-156.0637, 10)
  line L7 (-156.0637, 10) -> (-156.0637, 215)
  line L8 (-156.0637, 215) -> (-166.0637, 215)
  line L9 (-169.5637, 225) -> (-169.5637, 15)
  line L10 (-169.5637, 15) -> (-300.8137, 15)
  line L11 (-300.8137, 15) -> (-300.8137, 225)
  line L12 (-314.3137, 225) -> (-304.3137, 225)
  line L13 (-304.3137, 225) -> (-304.3137, 215)
  line L14 (-304.3137, 215) -> (-314.3137, 215)
  line L15 (-314.3137, 215) -> (-314.3137, 225)
  line L16 (-166.0637, 215) -> (-166.0637, 225)
  line L17 (-166.0637, 225) -> (-169.5637, 225)
  dimension "d151" = 10
  dimension "d443" = 10
  constraint horizontal L12
  constraint vertical L13
  constraint horizontal L14
  constraint vertical L15
  constraint coincident L0.end L1.start
  measures "d151" distance of L0.end L12.end
  measures "d443" distance of L12 L14
extrude "Extrude35" add sketch "Sketch38" along normal blind 10 contours L0 L1 L12 L13 L14 L15 bodies 1
sketch "Sketch39" plane through (0, 0, 225) normal (0, 0, 1) x (-1, 0, 0)
  line L0 (-156.0637, -44.4866) -> (-169.5637, -44.4866)
  line L1 (-169.5637, -44.4866) -> (-169.5637, -57.9866)
  line L2 (-166.0637, -67.9866) -> (-156.0637, -67.9866)
  line L3 (-156.0637, -67.9866) -> (-156.0637, -44.4866)
  line L4 (-156.0637, -44.4866) -> (-156.0637, -57.9866)
  circle A0 centre (-162.8137, -51.2366) radius 3.5
  line L5 (-169.5637, -57.9866) -> (-166.0637, -57.9866)
  line L6 (-166.0637, -57.9866) -> (-166.0637, -67.9866)
  dimension "d158" = 7
  constraint vertical L4
  measures "d158" diameter of A0
extrude "Extrude36" cut sketch "Sketch39" against normal blind 6 contours A0 bodies 1
sketch "Sketch40" plane through (0, 0, 225) normal (0, 0, 1) x (-1, 0, 0)
  line L0 (-300.8137, -44.4866) -> (-314.3137, -44.4866)
  line L1 (-314.3137, -44.4866) -> (-314.3137, -67.9866)
  line L2 (-314.3137, -67.9866) -> (-304.3137, -67.9866)
  line L3 (-304.3137, -67.9866) -> (-304.3137, -57.9866)
  line L4 (-304.3137, -57.9866) -> (-300.8137, -57.9866)
  line L5 (-300.8137, -57.9866) -> (-300.8137, -44.4866)
  circle A0 centre (-307.5637, -51.2366) radius 3.5
  dimension "d162" = 7
  measures "d162" diameter of A0
extrude "Extrude37" cut sketch "Sketch40" against normal blind 6 contours A0 bodies 1
sketch "Sketch41" plane through (159.5637, 0, 0) normal (1, 0, 0) x (0, 1, 0)
  line L0 (-118.5134, 5) -> (-36.0134, 5)
  line L1 (-36.0134, 5) -> (-36.0134, 145)
  line L2 (-36.0134, 145) -> (-32.5134, 145)
  line L3 (-32.5134, 145) -> (-32.5134, 225)
  line L4 (-32.5134, 225) -> (-118.5134, 225)
  line L5 (-118.5134, 225) -> (-118.5134, 5)
  line L6 (-118.5134, 225) -> (-108.5134, 225)
  line L7 (-108.5134, 225) -> (-108.5134, 215)
  line L8 (-108.5134, 215) -> (-118.5134, 215)
  line L9 (-118.5134, 215) -> (-118.5134, 225)
  dimension "d165" = 10
  dimension "d166" = 10
  constraint horizontal L6
  constraint vertical L7
  constraint horizontal L8
  constraint vertical L9
  constraint coincident L4.end L5.start
  measures "d165" distance of L4.end L6.end
  measures "d166" distance of L4.end L8.end
extrude "Extrude38" add sketch "Sketch41" along normal blind 10 contours L4 L5 L6 L7 L8 L9 bodies 1
sketch "Sketch42" plane through (310.8137, 0, 0) normal (-1, 0, 0) x (0, -1, 0)
  line L0 (36.0134, 5) -> (118.5134, 5)
  line L1 (118.5134, 5) -> (118.5134, 225)
  line L2 (118.5134, 225) -> (32.5134, 225)
  line L3 (32.5134, 225) -> (32.5134, 145)
  line L4 (32.5134, 145) -> (36.0134, 145)
  line L5 (36.0134, 145) -> (36.0134, 5)
  line L6 (118.5134, 225) -> (108.5134, 225)
  line L7 (108.5134, 225) -> (108.5134, 215)
  line L8 (108.5134, 215) -> (118.5134, 215)
  line L9 (118.5134, 215) -> (118.5134, 225)
  dimension "d169" = 10
  dimension "d170" = 10
  constraint horizontal L6
  constraint vertical L7
  constraint horizontal L8
  constraint vertical L9
  constraint coincident L1.end L2.start
  measures "d169" distance of L1.end L6.end
  measures "d170" distance of L1.end L8.end
extrude "Extrude39" add sketch "Sketch42" along normal blind 10 contours L1 L2 L6 L7 L8 L9 bodies 1
sketch "Sketch43" plane through (0, 0, 225) normal (0, 0, 1) x (-1, 0, 0)
  line L0 (-310.8137, 32.5134) -> (-310.8137, 108.5134)
  line L1 (-310.8137, 108.5134) -> (-300.8137, 108.5134)
  line L2 (-300.8137, 108.5134) -> (-300.8137, 118.5134)
  line L3 (-300.8137, 118.5134) -> (-169.5637, 118.5134)
  line L4 (-169.5637, 118.5134) -> (-169.5637, 108.5134)
  line L5 (-169.5637, 108.5134) -> (-159.5637, 108.5134)
  line L6 (-159.5637, 108.5134) -> (-159.5637, 32.5134)
  line L7 (-159.5637, 32.5134) -> (-156.0637, 32.5134)
  line L8 (-156.0637, 32.5134) -> (-156.0637, 122.0134)
  line L9 (-156.0637, 122.0134) -> (-314.3137, 122.0134)
  line L10 (-314.3137, 122.0134) -> (-314.3137, 32.5134)
  line L11 (-314.3137, 32.5134) -> (-310.8137, 32.5134)
  circle A0 centre (-162.8137, 115.2634) radius 3.5
  dimension "d173" = 7
  dimension "d411" = 6.75
  measures "d173" diameter of A0
  measures "d411" distance of L9 A0.centre
extrude "Extrude40" cut sketch "Sketch43" against normal blind 6 contours A0 bodies 1
sketch "Sketch44" plane through (0, 0, 225) normal (0, 0, 1) x (-1, 0, 0)
  line L0 (-310.8137, 32.5134) -> (-310.8137, 108.5134)
  line L1 (-310.8137, 108.5134) -> (-300.8137, 108.5134)
  line L2 (-300.8137, 108.5134) -> (-300.8137, 118.5134)
  line L3 (-300.8137, 118.5134) -> (-169.5637, 118.5134)
  line L4 (-169.5637, 118.5134) -> (-169.5637, 108.5134)
  line L5 (-169.5637, 108.5134) -> (-159.5637, 108.5134)
  line L6 (-159.5637, 108.5134) -> (-159.5637, 32.5134)
  line L7 (-159.5637, 32.5134) -> (-156.0637, 32.5134)
  line L8 (-156.0637, 32.5134) -> (-156.0637, 122.0134)
  line L9 (-156.0637, 122.0134) -> (-314.3137, 122.0134)
  line L10 (-314.3137, 122.0134) -> (-314.3137, 32.5134)
  line L11 (-314.3137, 32.5134) -> (-310.8137, 32.5134)
  line L12 (-314.3137, 122.0134) -> (-275.8657, 122.0134)
  line L13 (-314.3137, 72.5134) -> (-314.3137, 122.0134)
  circle A0 centre (-307.5637, 115.2634) radius 3.5
  circle A1 centre (-162.8137, 115.2634) radius 3.5
  dimension "d176" = 7
  dimension "d409" = 6.75
  dimension "d410" = 6.75
  constraint horizontal L12
  constraint vertical L13
  constraint coincident L9.end L10.start
  measures "d176" diameter of A0
  measures "d409" distance of L13 A0.centre
  measures "d410" distance of L12 A0.centre
extrude "Extrude41" cut sketch "Sketch44" against normal blind 6 contours A0 bodies 1
sketch "Sketch45" plane through (0, 0, 3) normal (0, 0, 1) x (-1, 0, 0)
  line L0 (-17.7235, -83.5) -> (106.5265, -83.5)
  line L1 (106.5265, -83.5) -> (106.5265, -73)
  line L2 (106.5265, -73) -> (116.5265, -73)
  line L3 (116.5265, -73) -> (116.5265, 0)
  line L4 (116.5265, 0) -> (120.0265, 0)
  line L5 (120.0265, 0) -> (120.0265, -76.5)
  line L6 (120.0265, -76.5) -> (110.0265, -76.5)
  line L7 (110.0265, -76.5) -> (110.0265, -87)
  line L8 (110.0265, -87) -> (-21.2235, -87)
  line L9 (-21.2235, -87) -> (-21.2235, -76.5)
  line L10 (-21.2235, -76.5) -> (-31.2235, -76.5)
  line L11 (-31.2235, -76.5) -> (-31.2235, 0)
  line L12 (-31.2235, 0) -> (-27.7235, 0)
  line L13 (-27.7235, 0) -> (-27.7235, -73)
  line L14 (-27.7235, -73) -> (-17.7235, -73)
  line L15 (-17.7235, -73) -> (-17.7235, -83.5)
  line L16 (-5.7917, -72.9167) -> (-5.7917, -61.9167)
  line L17 (-5.7917, -61.9167) -> (22.9083, -61.9167)
  line L18 (22.9083, -61.9167) -> (22.9083, -72.9167)
  line L19 (22.9083, -72.9167) -> (-5.7917, -72.9167)
  circle A0 centre (78.4015, -15) radius 2.5
  circle A1 centre (78.4015, -45) radius 2.5
  circle A2 centre (59.4015, -15) radius 2.5
  circle A3 centre (59.4015, 15) radius 2.5
  circle A4 centre (59.4015, -45) radius 2.5
  line L20 (12.9015, 40) -> (12.9015, 81)
  line L21 (12.9015, 81) -> (75.9015, 81)
  line L22 (75.9015, 81) -> (75.9015, 40)
  line L23 (75.9015, 40) -> (12.9015, 40)
  line L24 (-34.7235, -90) -> (123.5265, -90)
  line L25 (123.5265, -90) -> (123.5265, 90)
  line L26 (123.5265, 90) -> (-34.7235, 90)
  line L27 (-34.7235, 90) -> (-34.7235, -90)
  line L28 (110.0265, 86.5) -> (110.0265, 76.5)
  line L29 (110.0265, 76.5) -> (120.0265, 76.5)
  line L30 (120.0265, 76.5) -> (120.0265, 5)
  line L31 (116.5265, 5) -> (116.5265, 73)
  line L32 (116.5265, 73) -> (106.5265, 73)
  line L33 (106.5265, 73) -> (106.5265, 83)
  line L34 (-21.2235, 86.5) -> (110.0265, 86.5)
  circle A5 centre (-27.9735, 83.25) radius 2.5
  line L35 (106.5265, 83) -> (-17.7235, 83)
  circle A6 centre (78.4015, 15) radius 2.5
  line L36 (-27.7235, 73) -> (-27.7235, 5)
  line L37 (-27.7235, 5) -> (-31.2235, 5)
  line L38 (-31.2235, 5) -> (-31.2235, 76.5)
  line L39 (-31.2235, 76.5) -> (-21.2235, 76.5)
  line L40 (-21.2235, 76.5) -> (-21.2235, 86.5)
  line L41 (-17.7235, 83) -> (-17.7235, 73)
  line L42 (-17.7235, 73) -> (-27.7235, 73)
  circle A7 centre (10.4015, -45) radius 2.5
  circle A8 centre (29.4015, 15) radius 2.5
  circle A9 centre (29.4015, -15) radius 2.5
  circle A10 centre (29.4015, -45) radius 2.5
  circle A11 centre (10.4015, 15) radius 2.5
  circle A12 centre (10.4015, -15) radius 2.5
  circle A13 centre (-4.7235, 40) radius 3.5
  line L43 (120.0265, 5) -> (116.5265, 5)
  dimension "d198" = 5
  dimension "d348" = 6.75
  dimension "d349" = 6.75
  measures "d198" diameter of A5
  measures "d348" distance of L27 A5.centre
  measures "d349" distance of L26 A5.centre
extrude "Extrude42" cut sketch "Sketch45" against normal blind 3 contours A5 bodies 2